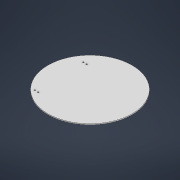
# Autodesk Inventor part: flame
Saved by Autodesk Inventor 2022 (Build 260153000, 153)
## iProperties
Created: 2021-09-22
Part Number: flame
Material: 一般
Document SubType Name: Modeling
Designer: shiok
Density: 1 g/cm^3
Appearance: 既定
Author: shiok
Autodesk Inventor part; units mm, degrees
ref_plane "YZ Plane" through (0, 0, 0) normal (1, 0, 0) x (0, 1, 0)
ref_plane "XZ Plane" through (0, 0, 0) normal (0, 1, 0) x (-1, 0, 0)
ref_plane "XY Plane" through (0, 0, 0) normal (0, 0, 1) x (1, 0, 0)
sketch "スケッチ1" plane through (0, 0, 0) normal (0, 1, 0) x (-1, 0, 0)
  circle A0 centre (0, 0) radius 62.5
  dimension "d41" = 125
  constraints: 1 centre point
  measures "d41" diameter of A0
extrude "押し出し1" add sketch "スケッチ1" along normal blind 1.35
sketch "スケッチ6" plane through (0, 1.35, 0) normal (0, 1, 0) x (1, 0, 0)
  line L0 (-40, -42) -> (-35, -42) construction
  line L1 (-35, -42) -> (-35, 30) construction
  line L2 (-35, 30) -> (-40, 30) construction
  line L3 (-40, 30) -> (-40, -42) construction
  line L4 (-35, 0) -> (-40, 0) construction
  line L5 (-42.5, 20) -> (-42.5, -20) construction
  line L6 (-40, -42) -> (-35, -42) construction
  line L7 (-35, -42) -> (-35, 30) construction
  line L8 (-35, 30) -> (-40, 30) construction
  line L9 (-40, 30) -> (-40, -42) construction
  line L10 (-35, 0) -> (-40, 0) construction
  line L11 (-42.5, 20) -> (-42.5, -20) construction
  point P0 (0, 0)
  dimension "d52" = 5
  dimension "d53" = 72
  dimension "d54" = 30
  dimension "d55" = 2.5
  dimension "d56" = 5
  dimension "d57" = 72
  dimension "d58" = 30
  dimension "d59" = 2.5
  constraints: 24 end point, 4 parallel, 4 perpendicular, 4 point on line, 2 horizontal
  measures "d52" distance of L2.end L1.end
  measures "d53" distance of L1.end L0.end
  measures "d54" distance between parallel lines of L2 L4
  measures "d55" distance between parallel lines of L3 L5
  measures "d56" distance of L8.end L7.end
  measures "d57" distance of L7.end L6.end
  measures "d58" distance between parallel lines of L8 L10
  measures "d59" distance between parallel lines of L9 L11
hole "穴3" at (-35, 1.35, -30) at (-40, 1.35, -30) at (-40, 1.35, 42) at (-35, 1.35, 42) direction (0, -1, 0) diameter 2.013 end through all thread size "M2.5x0.45" class "6H" standard "ISO Metric profile"
